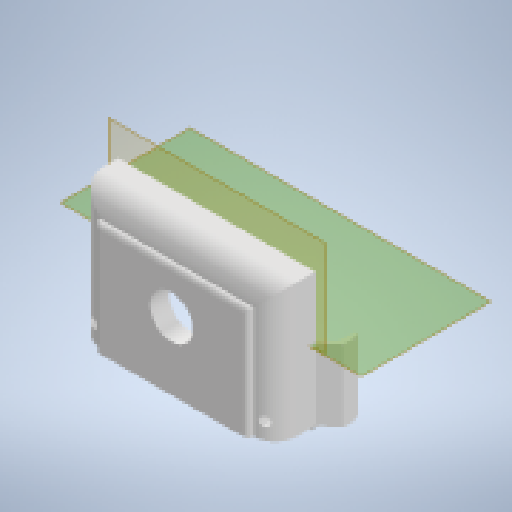
# Autodesk Inventor part: крышка камера
Saved by Autodesk Inventor 2024.2 (Build 282272000, 272)
## iProperties
Created: 2025-10-05
Part Number: крышка камера
Material: Типовые
Document SubType Name: Modeling
Designer: katya_notebook
Density: 1 g/cm^3
Appearance: По умолчанию
Author: katya_notebook
Autodesk Inventor part; units mm, degrees
ref_plane "YZ Plane" through (0, 0, 0) normal (1, 0, 0) x (0, 1, 0)
ref_plane "XZ Plane" through (0, 0, 0) normal (0, 1, 0) x (-1, 0, 0)
ref_plane "XY Plane" through (0, 0, 0) normal (0, 0, 1) x (1, 0, 0)
ref_plane "РабПлоскость1" through (0, 0, 0) normal (0, 0, 1) x (1, 0, 0)
sketch "Эскиз1" plane through (0, 0, 0) normal (0, 0, 1) x (1, 0, 0)
  line L0 (53.699145, 17.53431) -> (19.699145, 17.53431)
  line L1 (0, 17.53431) -> (0, -26.68)
  line L2 (0, -26.68) -> (73.399146, -26.68)
  line L3 (73.399146, 17.53431) -> (73.399146, -26.68)
  line L4 (0, 17.53431) -> (0, 23.022859)
  line L5 (73.399146, 17.53431) -> (73.399146, 23.022859)
  line L6 (73.399146, 23.022859) -> (0, 23.022859)
  line L7 (71.28909, -13.500049) -> (71.28909, 13.499954)
  constraints: 12 end point, 2 perpendicular, 1 horizontal, 1 vertical
extrude "Выдавливание1" add sketch "Эскиз1" along normal blind 15
sketch "Эскиз2" plane through (0, 0, 0) normal (0, 0, -1) x (-1, 0, 0)
  point P0 (0, 0)
sketch "Эскиз3" plane through (0, 0, 0) normal (0, 0, 1) x (1, 0, 0)
  circle A0 centre (36.699145, -1.46569) radius 8
  line L0 (53.699145, 17.53431) -> (19.699145, 17.53431)
  line L1 (19.699145, -20.46569) -> (53.699145, -20.46569)
  line L2 (17.699145, 15.53431) -> (17.699145, -18.46569)
  line L3 (55.699145, -18.46569) -> (55.699145, 15.53431)
  line L4 (57.699145, 19.53431) -> (15.699145, 19.53431)
  line L5 (15.699145, 19.53431) -> (15.699145, -22.46569)
  line L6 (15.699145, -22.46569) -> (57.699145, -22.46569)
  line L7 (57.699145, -22.46569) -> (57.699145, 19.53431)
  line L8 (57.699145, 19.53431) -> (15.699145, -22.46569) construction
  line L9 (15.699145, 19.53431) -> (57.699145, -22.46569) construction
  point P0 (0, 0)
  dimension "d2" = 42
  dimension "d3" = 42
  constraints: 12 end point, 2 midpoint, 2 parallel, 1 horizontal, 1 perpendicular
  measures "d2" distance of L6.end L5.end
  measures "d3" distance of L4.start L6.end
extrude "Выдавливание2" cut sketch "Эскиз3" along normal blind 15
sketch "Эскиз4" plane through (36.699145, -1.46569, 15) normal (0, 0, 1) x (1, 0, 0)
  circle A0 centre (0, 0) radius 8
  point P0 (-36.699145, 1.46569)
  dimension "d8" = 16
  constraints: 1 centre point
  measures "d8" diameter of A0
extrude "Выдавливание3" cut sketch "Эскиз4" against normal blind 15
sketch "Эскиз5" plane through (0, 0, 15) normal (0, 0, 1) x (1, 0, 0)
  line L0 (15.699145, 19.53431) -> (57.699145, 19.53431)
  line L1 (15.699145, -22.46569) -> (15.699145, 19.53431)
  line L2 (15.699145, 19.53431) -> (57.699145, 19.53431)
  line L3 (57.699145, 19.53431) -> (57.699145, -22.46569)
  line L4 (57.699145, -22.46569) -> (15.699145, -22.46569)
  line L5 (15.699145, -22.46569) -> (15.699145, 19.53431)
  circle A0 centre (36.699145, -1.46569) radius 8
  circle A1 centre (36.699145, -1.46569) radius 8
  point P0 (0, 0)
  constraints: 8 end point, 2 parallel, 1 centre point, 1 coincident, 1 concentric, 1 horizontal, 1 perpendicular
extrude "Выдавливание4" add sketch "Эскиз5" against normal blind 5
sketch "Эскиз6" plane through (0, 0, 15) normal (0, 0, 1) x (1, 0, 0)
  circle A0 centre (4.859145, -20.52069) radius 1.7
  circle A1 centre (68.649145, -20.52069) radius 1.7
  point P0 (0, 0)
extrude "Выдавливание5" cut sketch "Эскиз6" against normal blind 15
ref_plane "РабПлоскость2" through (83.299145, 0, -26.484913) normal (0, -1, 0) x (-1, 0, 0)
sketch "Эскиз7" plane through (83.299145, 0, -26.484913) normal (0, -1, 0) x (-1, 0, 0)
  line L0 (86.92, -21.657107) -> (83.299145, -26.484913)
  line L1 (86.92, -17.442893) -> (86.92, -21.657107)
  line L2 (91.12, -17.442893) -> (86.92, -17.442893)
  line L3 (83.299145, -26.484913) -> (86.92, -21.657107)
  line L4 (86.92, -21.657107) -> (86.92, -17.442893)
  line L5 (88.2462, -17.442893) -> (86.92, -17.442893)
  line L6 (88.2462, -17.442893) -> (88.2462, -15.442893)
  line L7 (88.2462, -15.442893) -> (87.109572, -15.442893)
  line L8 (87.109572, -15.442893) -> (85.109572, -15.442893)
  line L9 (83.299145, -26.484913) -> (81.299145, -26.484913)
  line L10 (9.899999, -26.484913) -> (83.299145, -26.484913)
  line L11 (88.92, -21.657107) -> (88.92, -15.442893)
  line L12 (88.92, -15.442893) -> (85.109572, -15.442893)
  line L13 (88.92, -21.657107) -> (81.299145, -26.484913)
  line L14 (46.6, -4.827665) -> (46.6, -53.254819)
  line L15 (6.28, -21.657107) -> (9.900855, -26.484913)
  line L16 (6.28, -17.442893) -> (6.28, -21.657107)
  line L17 (9.900855, -26.484913) -> (6.28, -21.657107)
  line L18 (6.28, -21.657107) -> (6.28, -17.442893)
  line L19 (4.9538, -17.442893) -> (6.28, -17.442893)
  line L20 (4.9538, -17.442893) -> (4.9538, -15.442893)
  line L21 (4.9538, -15.442893) -> (6.090428, -15.442893)
  line L22 (6.090428, -15.442893) -> (8.090428, -15.442893)
  line L23 (9.900855, -26.484913) -> (11.900855, -26.484913)
  line L24 (4.28, -21.657107) -> (4.28, -15.442893)
  line L25 (4.28, -15.442893) -> (8.090428, -15.442893)
  line L26 (4.28, -21.657107) -> (11.900855, -26.484913)
  point P0 (87.030057, -15.442893)
  point P1 (85.109572, -24.07101)
  dimension "d13" = 2
  dimension "d14" = 2
  dimension "d15" = 2
  dimension "d16" = 2
  constraints: 46 end point, 10 symmetric about line, 3 vertical, 2 collinear, 2 horizontal, 2 perpendicular, 2 point on line
  measures "d13" distance of L6.end L5.start
  measures "d14" distance of L8.end L7.end
  measures "d15" distance of L0.end L9.end
  measures "d16" distance of L11.start L0.start
ref_plane "РабПлоскость3" through (-3.000855, -24.18, -16.427807) normal (0.7071068, 0.7071068, 0) x (-0.7071068, 0.7071068, 0)
extrude "Выдавливание6" add sketch "Эскиз7" along normal up to surface contours L0 L9 L13 surface through (-3.000855, -24.18, -16.427807) normal (0.7071068, 0.7071068, 0)
ref_plane "РабПлоскость4" through (83.299145, 0, -26.484913) normal (0, -1, 0) x (-1, 0, 0)
sketch "Эскиз8" plane through (83.299145, 0, -26.484913) normal (0, -1, 0) x (-1, 0, 0)
  line L0 (6.28, -18.260908) -> (9.900855, -26.484913)
  line L1 (9.900855, -26.484913) -> (11.885639, -26.484913)
  line L2 (9.899999, -26.484913) -> (83.299145, -26.484913)
  line L3 (6.28, -9.442893) -> (6.28, -18.260908)
  line L4 (4.28, -21.657107) -> (11.900855, -26.484913)
  line L5 (11.900855, -26.484913) -> (4.28, -21.657107)
  line L6 (4.28, -21.657107) -> (4.28, -15.442893)
  line L7 (4.9538, -17.442893) -> (6.28, -17.442893)
  line L8 (4.9538, -17.442893) -> (4.9538, -15.442893)
  line L9 (4.9538, -15.442893) -> (6.090428, -15.442893)
  line L10 (4.9538, -17.442893) -> (4.9538, -15.442893)
  line L11 (4.28, -21.657107) -> (4.28, -15.442893)
  line L12 (4.9538, -15.442893) -> (4.28, -15.442893)
  line L13 (4.9538, -17.442893) -> (6.28, -17.442893)
  point P0 (6.28, -15.442893)
  point P1 (6.28, -17.442893)
  point P2 (9.127252, -24.727838)
  constraints: 16 end point, 2 horizontal, 2 point on line, 2 vertical, 1 perpendicular, 1 other
ref_plane "РабПлоскость5" through (73.899145, -26.68, -16.427807) normal (-0.7071068, 0.7071068, 0) x (0, 0, 1)
extrude "Выдавливание7" add sketch "Эскиз8" along normal up to surface contours L4 L2 L1 L0 surface through (73.899145, -26.68, -16.427807) normal (-0.7071068, 0.7071068, 0)
fillet "Сопряжение2" radius 8 3 edges at (0, -1.8286, 15) (36.6996, 23.0229, 15) (73.3991, -1.8286, 15)
sketch "Эскиз9" plane through (0, 0, 10) normal (0, 0, -1) x (-1, 0, 0)
  circle A0 centre (-36.699145, -1.46569) radius 8
  line L0 (-22.199145, -15.96569) -> (-51.199145, -15.96569)
  line L1 (-51.199145, -15.96569) -> (-51.199145, 13.03431)
  line L2 (-51.199145, 13.03431) -> (-22.199145, 13.03431)
  line L3 (-22.199145, 13.03431) -> (-22.199145, -15.96569)
  line L4 (-22.199145, -15.96569) -> (-51.199145, 13.03431) construction
  line L5 (-51.199145, -15.96569) -> (-22.199145, 13.03431) construction
  circle A1 centre (-51.199145, 13.03431) radius 2.1
  circle A2 centre (-51.199145, -15.96569) radius 2.1
  circle A3 centre (-22.199145, 13.03431) radius 2.1
  circle A4 centre (-22.199145, -15.96569) radius 2.1
  point P0 (0, 0)
  dimension "d23" = 29
  dimension "d24" = 4.2
  constraints: 12 end point, 4 centre point, 4 coincident, 3 equal radius, 2 midpoint, 2 parallel, 2 perpendicular, 1 horizontal
  measures "d23" distance of L1.end L2.end
  measures "d24" diameter of A4
extrude "Выдавливание8" cut sketch "Эскиз9" against normal blind 5 contours A2 L1 L0 | L0 L1 A2 | A4 L3 L0 | L0 L3 A4 | A1 L2 L1 | L1 L2 A1 | A3 L2 L3 | L3 L2 A3
sketch "Эскиз10" plane through (0, 0, 15) normal (0, 0, 1) x (1, 0, 0)
  arc A0 (21.524108, 15.022859) -> (22.874182, 15.022859) centre (22.199145, 13.03431) ccw
  line L0 (8, 15.022859) -> (21.524108, 15.022859)
  line L1 (8, -26.68) -> (8, 15.022859)
  line L2 (65.399146, 15.022859) -> (65.399146, -26.68)
  line L3 (51.874182, 15.022859) -> (65.399146, 15.022859)
  arc A1 (50.524108, 15.022859) -> (51.874182, 15.022859) centre (51.199145, 13.03431) ccw
  line L4 (22.874182, 15.022859) -> (50.524108, 15.022859)
  circle A2 centre (36.699145, -1.46569) radius 8
  circle A3 centre (22.199145, -15.96569) radius 2.1
  circle A4 centre (51.199145, -15.96569) radius 2.1
  spline S0 degree 5 poles (21.524108, 15.022859) (21.656302, 15.067734) (21.790679, 15.101099) (21.92639, 15.123239) (22.062764, 15.13431) (22.335526, 15.13431) (22.4719, 15.123239) (22.607611, 15.101099) (22.741988, 15.067733) (22.874182, 15.022859) knots 0 0 0 0 0 0 0.50000012 0.50000012 0.50000012 0.50000012 1 1 1 1 1 1
  spline S1 degree 5 poles (50.524108, 15.022859) (50.656302, 15.067734) (50.790679, 15.101099) (50.92639, 15.123239) (51.062764, 15.13431) (51.335526, 15.13431) (51.4719, 15.123239) (51.607611, 15.101099) (51.741988, 15.067733) (51.874182, 15.022859) knots 0 0 0 0 0 0 0.50000012 0.50000012 0.50000012 0.50000012 1 1 1 1 1 1
  line L5 (8, -26.68) -> (65.399146, -26.68)
  point P0 (0, 0)
  constraints: 2 horizontal alignment
extrude "Выдавливание9" add sketch "Эскиз10" along normal blind 2 contours S0 A0 | A0 L4 A1 L3 L2 L5 L1 L0 | S1 A1 | A3 | A4
fillet "Сопряжение3" radius 20 4 edges at (21.5241, 15.0229, 16) (22.8742, 15.0229, 16) (51.8742, 15.0229, 16) (50.5241, 15.0229, 16)
fillet "Сопряжение4" radius 2 11 edges at (59.4075, 15.0229, 17) (51.1991, 15.1343, 17) (49.9867, 15.0481, 17) (36.6991, 15.0229, 17) (23.4115, 15.0481, 17) (22.1991, 15.1343, 17) (20.9867, 15.0481, 17) (13.9912, 15.0229, 17) (52.4115, 15.0481, 17) (65.3991, -5.8286, 17) (8, -5.8286, 17)
sketch "Эскиз11" plane through (0, 0, 0) normal (0, 0, -1) x (-1, 0, 0)
  spline S0 degree 3 poles (-65.089088, 2.701898) (-65.160681, 2.584918) (-65.245795, 2.478306) (-65.490008, 2.23445) (-65.682611, 2.103422) (-66.102007, 1.930885) (-66.328709, 1.88931) (-66.758463, 1.88931) (-66.989383, 1.934137) (-67.41102, 2.112117) (-67.601938, 2.245146) (-67.897436, 2.546451) (-68.024932, 2.733515) (-68.195829, 3.147354) (-68.239088, 3.374358) (-68.239088, 3.804263) (-68.195829, 4.031267) (-68.024932, 4.445105) (-67.897436, 4.63217) (-67.601938, 4.933475) (-67.41102, 5.066503) (-66.989383, 5.244483) (-66.758463, 5.28931) (-66.328709, 5.28931) (-66.102007, 5.247736) (-65.682611, 5.075198) (-65.490008, 4.94417) (-65.245795, 4.700314) (-65.160681, 4.593703) (-65.089088, 4.476722) knots 0.08916697 0.08916697 0.08916697 0.08916697 0.12822187 0.12822187 0.19273489 0.19273489 0.25724792 0.25724792 0.32451938 0.32451938 0.39179083 0.39179083 0.4562766 0.4562766 0.52076237 0.52076237 0.58524814 0.58524814 0.64973391 0.64973391 0.71700537 0.71700537 0.78427683 0.78427683 0.84878985 0.84878985 0.91330288 0.91330288 0.95235778 0.95235778 0.95235778 0.95235778
  arc A0 (-65.089088, 2.701898) -> (-65.089088, 4.476722) centre (-66.539088, 3.58931) ccw
  spline S1 degree 3 poles (-4.089088, 4.635446) (-4.045336, 4.691489) (-3.99862, 4.744035) (-3.798092, 4.944174) (-3.605736, 5.075086) (-3.186533, 5.247628) (-2.959763, 5.28931) (-2.530165, 5.28931) (-2.299533, 5.244648) (-1.878272, 5.06712) (-1.687452, 4.934372) (-1.39141, 4.633176) (-1.263553, 4.445723) (-1.092327, 4.031347) (-1.049088, 3.804211) (-1.049088, 3.58931) (-1.049088, 3.374409) (-1.092327, 3.147273) (-1.263553, 2.732898) (-1.39141, 2.545444) (-1.687452, 2.244248) (-1.878272, 2.1115) (-2.299533, 1.933972) (-2.530165, 1.88931) (-2.959763, 1.88931) (-3.186533, 1.930992) (-3.605736, 2.103534) (-3.798092, 2.234447) (-3.99862, 2.434585) (-4.045336, 2.487131) (-4.089088, 2.543174) knots -0.41216506 -0.41216506 -0.41216506 -0.41216506 -0.3915556 -0.3915556 -0.32716248 -0.32716248 -0.26276936 -0.26276936 -0.19585496 -0.19585496 -0.12894057 -0.12894057 -0.06447028 -0.06447028 0 0 0 0.06447028 0.06447028 0.12894057 0.12894057 0.19585496 0.19585496 0.26276936 0.26276936 0.32716248 0.32716248 0.3915556 0.3915556 0.41216506 0.41216506 0.41216506 0.41216506
  arc A1 (-4.089088, 4.635446) -> (-4.089088, 2.543174) centre (-2.749088, 3.58931) ccw
  line L0 (-2.749088, 3.58931) -> (-4.859088, 3.58931)
  circle A2 centre (-4.859088, 3.58931) radius 2.1
  line L1 (-66.539088, 3.58931) -> (-64.429088, 3.58931)
  circle A3 centre (-64.429088, 3.58931) radius 2.1
  point P0 (0, 0)
  dimension "d38" = 2.11
  dimension "d39" = 4.2
  constraints: 4 end point, 3 coincident, 2 centre point, 2 horizontal, 1 collinear, 1 equal radius
  measures "d38" distance of L0.start L0.end
  measures "d39" diameter of A2
extrude "Выдавливание10" cut sketch "Эскиз11" against normal blind 5 contours A0 S0 A3 | S0 A3 L1 A0 | L1 A3 S0 A0 | A1 S1 A2 | S1 A2 L0 A1 | L0 A2 S1 A1
sketch "Эскиз12" plane through (0, -26.68, 0) normal (0, -1, 0) x (1, 0, 0)
  line L0 (-1.810428, -2.413903) -> (2, 0)
  line L1 (2, 0) -> (0, 0)
  line L2 (0, 0) -> (-1.810428, -2.413903)
  line L3 (10, 17) -> (63.399146, 17)
  line L4 (36.699573, 17) -> (36.699573, -97.462231)
  line L5 (78.346201, -9.04202) -> (78.346201, -11.04202)
  line L6 (78.346201, -11.04202) -> (77.130058, -11.04202)
  line L7 (77.130058, -11.04202) -> (77.130058, -4.827807)
  line L8 (77.130058, -4.827807) -> (71.399146, 0)
  line L9 (71.399146, 0) -> (73.399146, 0)
  line L10 (73.399146, 0) -> (79.130058, -4.827807)
  line L11 (79.130058, -4.827807) -> (79.130058, -9.04202)
  line L12 (79.130058, -9.04202) -> (78.346201, -9.04202)
  constraints: 18 end point, 3 symmetric about line, 1 midpoint, 1 vertical
ref_plane "РабПлоскость6" through (-16.708271, 0, -45.649594) normal (0, -1, 0) x (1, 0, 0)
extrude "Выдавливание11" add sketch "Эскиз12" against normal up to surface (26.68 mm away) contours L5 L6 L7 L8 L9 L10 L11 L12
sketch "Эскиз13" plane through (2, -26.68, 0) normal (0, -1, 0) x (1, 0, 0)
  line L0 (71.899145, -2.174038) -> (69.144378, -2.174038)
  line L1 (69.144378, -2.174038) -> (69.144378, 0.339814)
  line L2 (69.144378, 0.339814) -> (71.899145, 0.339814)
  line L3 (71.899145, 0.339814) -> (71.899145, -2.174038)
  point P0 (-2, 0)
  constraints: 8 end point, 2 parallel, 1 horizontal, 1 perpendicular
extrude "Выдавливание12" cut sketch "Эскиз13" along normal blind 10
sketch "Эскиз14" plane through (0, 0, 0) normal (0, 0, -1) x (-1, 0, 0)
  spline S0 degree 3 poles (-6.199145, 4.635446) (-6.155392, 4.691489) (-6.108676, 4.744035) (-5.908148, 4.944174) (-5.715793, 5.075086) (-5.296589, 5.247628) (-5.069819, 5.28931) (-4.640222, 5.28931) (-4.409589, 5.244648) (-3.988329, 5.06712) (-3.797508, 4.934372) (-3.501467, 4.633176) (-3.37361, 4.445723) (-3.202383, 4.031347) (-3.159145, 3.804211) (-3.159145, 3.58931) (-3.159145, 3.374409) (-3.202383, 3.147273) (-3.37361, 2.732898) (-3.501467, 2.545444) (-3.797508, 2.244248) (-3.988329, 2.1115) (-4.409589, 1.933972) (-4.640222, 1.88931) (-5.069819, 1.88931) (-5.296589, 1.930992) (-5.715793, 2.103534) (-5.908148, 2.234447) (-6.108676, 2.434585) (-6.155392, 2.487131) (-6.199145, 2.543174) knots -0.41216506 -0.41216506 -0.41216506 -0.41216506 -0.3915556 -0.3915556 -0.32716248 -0.32716248 -0.26276936 -0.26276936 -0.19585496 -0.19585496 -0.12894057 -0.12894057 -0.06447028 -0.06447028 0 0 0 0.06447028 0.06447028 0.12894057 0.12894057 0.19585496 0.19585496 0.26276936 0.26276936 0.32716248 0.32716248 0.3915556 0.3915556 0.41216506 0.41216506 0.41216506 0.41216506
  spline S1 degree 3 poles (-67.199145, 2.701898) (-67.270738, 2.584918) (-67.355852, 2.478306) (-67.600065, 2.23445) (-67.792668, 2.103422) (-68.212064, 1.930885) (-68.438766, 1.88931) (-68.86852, 1.88931) (-69.09944, 1.934137) (-69.521076, 2.112117) (-69.711995, 2.245146) (-70.007492, 2.546451) (-70.134989, 2.733515) (-70.305886, 3.147354) (-70.349145, 3.374358) (-70.349145, 3.804263) (-70.305886, 4.031267) (-70.134989, 4.445105) (-70.007492, 4.63217) (-69.711995, 4.933475) (-69.521076, 5.066503) (-69.09944, 5.244483) (-68.86852, 5.28931) (-68.438766, 5.28931) (-68.212064, 5.247736) (-67.792668, 5.075198) (-67.600065, 4.94417) (-67.355852, 4.700314) (-67.270738, 4.593703) (-67.199145, 4.476722) knots 0.08916697 0.08916697 0.08916697 0.08916697 0.12822187 0.12822187 0.19273489 0.19273489 0.25724792 0.25724792 0.32451938 0.32451938 0.39179083 0.39179083 0.4562766 0.4562766 0.52076237 0.52076237 0.58524814 0.58524814 0.64973391 0.64973391 0.71700537 0.71700537 0.78427683 0.78427683 0.84878985 0.84878985 0.91330288 0.91330288 0.95235778 0.95235778 0.95235778 0.95235778
  arc A0 (-6.199145, 4.635446) -> (-6.199145, 2.543174) centre (-4.859145, 3.58931) ccw
  arc A1 (-67.199145, 2.701898) -> (-67.199145, 4.476722) centre (-68.649145, 3.58931) ccw
  point P0 (0, 0)
